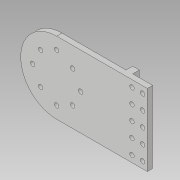
# Autodesk Inventor part: dynamixel_pro_frame_part3
Saved by Autodesk Inventor 2017 (Build 210142000, 142)
## iProperties
Part Number: dynamixel_pro_frame_part3
Material: Generisch
Document SubType Name: Modeling
Designer: Max
Density: 1 g/cm^3
Appearance: Vorgabe
Author: Max
Autodesk Inventor part; units mm, degrees
ref_plane "YZ Plane" through (0, 0, 0) normal (1, 0, 0) x (0, 1, 0)
ref_plane "XZ Plane" through (0, 0, 0) normal (0, 1, 0) x (-1, 0, 0)
ref_plane "XY Plane" through (0, 0, 0) normal (0, 0, 1) x (1, 0, 0)
sketch "Skizze1" plane through (0, 0, 0) normal (0, 1, 0) x (-1, 0, 0)
  line L0 (-50, 27) -> (50, 27)
  line L1 (50, 27) -> (50, -27) construction
  line L2 (50, -27) -> (-50, -27)
  line L3 (-50, -27) -> (-50, 27)
  line L4 (-50, 27) -> (50, -27) construction
  line L5 (50, 27) -> (-50, -27) construction
  line L6 (0, 0) -> (66.4326, 0) construction
  arc A0 (18, -27) -> (18, 27) centre (18, 0) ccw
  dimension "d0" = 54
  dimension "d1" = 100
  dimension "d12" = 68
  dimension "d13" = 90
  constraints: 14 end point, 3 point on line, 2 horizontal, 2 midpoint, 2 parallel, 2 point on circle, 1 centre point, 1 perpendicular
  measures "d0" distance of L2.end L0.start
  measures "d1" distance of L1.end L2.end
  measures "d12" distance from line of A0.centre L3
extrude "Extrusion1" add sketch "Skizze1" along normal blind 4
sketch "Skizze5" plane through (0, 4, 0) normal (0, 1, 0) x (1, 0, 0)
  line L0 (-18, -27) -> (50, -27) projected
  line L1 (50, -27) -> (50, 27) projected
  line L2 (50, 27) -> (-18, 27) projected
  arc A0 (-18, 27) -> (-18, -27) centre (-18, 0) ccw projected
  line L3 (35, -27) -> (30, -27)
  line L4 (30, -27) -> (30, 27)
  line L5 (30, 27) -> (35, 27)
  line L6 (35, 27) -> (35, -27)
  point P0 (0, 0)
  dimension "d14" = 15
  dimension "d15" = 5
  constraints: 8 end point, 2 parallel, 2 point on line, 1 horizontal, 1 perpendicular
  measures "d14" distance between parallel lines of L6 L1
  measures "d15" distance between parallel lines of L4 L6
extrude "Extrusion4" add sketch "Skizze5" along normal blind 5 contours L4 L2 L6 L0
sketch "Skizze6" plane through (0, 4, 0) normal (0, 1, 0) x (1, 0, 0)
  line L0 (35, 27) -> (35, -27) projected
  line L1 (35, -27) -> (50, -27) projected
  line L2 (50, -27) -> (50, 27) projected
  line L3 (50, 27) -> (35, 27) projected
  line L4 (0, 0) -> (67.4565, 0) construction
  point P0 (46.5, 0)
  dimension "d18" = 3.5
  constraints: 2 end point, 1 horizontal, 1 point on line
  measures "d18" distance from line of point (46.5, 0) L2
hole "Bohrung1" at (46.5, 4, 0) direction (0, -1, 0) diameter 3.4 end through all clearance for "Inbusschraube ISO 4762" size "M3" standard "ISO"
pattern_linear "Rechteckige Anordnung1" count 5 spacing 11 along (0, 0, -1) count 2 spacing 8 along (-1, 0, 0) of "Bohrung1" first direction both ways yes
sketch "Skizze7" plane through (0, 0, 0) normal (0, -1, 0) x (1, 0, 0)
  arc A0 (-18, 27) -> (-18, -27) centre (-18, 0) ccw projected
  line L0 (-6, 12) -> (-30, 12)
  line L1 (-30, 12) -> (-30, -12)
  line L2 (-30, -12) -> (-6, -12)
  line L3 (-6, -12) -> (-6, 12)
  line L4 (-6, 12) -> (-30, -12) construction
  line L5 (-36, 18) -> (0, -18) construction
  circle A1 centre (-18, 0) radius 18
  line L6 (-18, 22.4057) -> (-18, -22.4722) construction
  line L7 (3.1609, 0) -> (-39.488, 0) construction
  point P0 (0, 0)
  point P1 (-18, -18)
  point P2 (-36, 0)
  point P3 (-18, 18)
  point P4 (0, 0)
  dimension "d32" = 24
  dimension "d33" = 24
  dimension "d35" = 36
  constraints: 16 end point, 4 point on line, 3 midpoint, 3 point on circle, 2 coincident, 2 horizontal, 2 parallel, 1 centre point, 1 perpendicular, 1 vertical
  measures "d32" distance of L1.end L2.end
  measures "d33" distance of L0.end L1.end
  measures "d35" diameter of A1
hole "Bohrung2" at (-18, 0, -18) at (-36, 0, 0) at (-18, 0, 18) at (0, 0, 0) at (-6, 0, -12) at (-30, 0, -12) at (-30, 0, 12) at (-6, 0, 12) direction (0, 1, 0) diameter 3.4 end through all clearance for "Inbusschraube ISO 4762" size "M3" standard "ISO"
